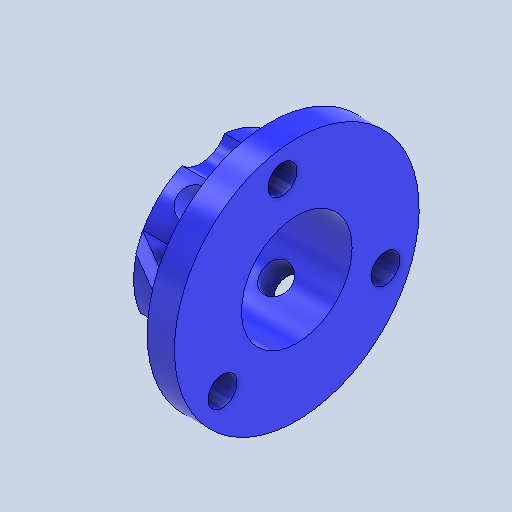
# Autodesk Inventor part: install-encoder-v1-3DP-Shaft-F
Saved by Autodesk Inventor 2025.2 (Build 292293000, 293)
## iProperties
Created: 2024-02-12
Part Number: install-encoder-v1-3DP-Shaft-F
Material: ABS プラスチック
Document SubType Name: Modeling
Designer: haruy
Density: 1.06 g/cm^3
Appearance: 青 - 壁塗料 - 光沢
Author: haruy
Autodesk Inventor part; units mm, degrees
sketch "スケッチ1" plane through (0, 0, 0) normal (1, 0, 0) x (0, 1, 0)
  circle A0 centre (0, 0) radius 13.5
  circle A1 centre (0, 0) radius 6.1
  circle A2 centre (0, 0) radius 10.5
  circle A3 centre (10.3803, 1.5811) radius 1.6
  circle A4 centre (-6.5594, 8.199) radius 1.6
  circle A5 centre (-3.8208, -9.7801) radius 1.6
  circle A6 centre (0, 0) radius 9
  circle A7 centre (-6.5594, 8.199) radius 3
  circle A8 centre (10.3803, 1.5811) radius 3
  circle A9 centre (-3.8208, -9.7801) radius 3
  line L0 (0, 0) -> (8.4336, -10.5416)
  line L1 (4.8067, -7.6089) -> (7.6295, -11.1373)
  line L2 (6.3684, -6.3595) -> (9.1913, -9.8879)
  line L3 (0, 0) -> (10.3803, 1.5811)
  line L4 (0, 0) -> (-2.0329, 13.3461)
  line L5 (0, 0) -> (-3.8208, -9.7801)
  line L6 (0, 0) -> (-12.5745, 4.9125)
  point P0 (-5.3784, -7.2162)
  point P1 (-0.9377, -8.951)
  point P2 (8.9386, -1.0497)
  point P3 (8.2206, 3.6635)
  point P4 (-3.5602, 8.2659)
  point P5 (-7.283, 5.2876)
  dimension "d2" = 21
  dimension "d0" = 27
  dimension "d1" = 12.2
  dimension "d3" = 3.2
  dimension "d6" = 360
  dimension "d10" = 18
  dimension "d11" = 6
  dimension "d12" = 6
  dimension "d13" = 6
  dimension "d17" = 60
  dimension "d18" = 1
  dimension "d19" = 1
  dimension "d32" = 90
  dimension "d33" = 90
  constraints: 14 end point, 9 centre point, 7 coincident, 7 point on circle, 2 parallel, 10 other
  measures "d0" diameter of A0
  measures "d1" diameter of A1
  measures "d3" diameter of A3
  measures "d10" diameter of A6
  measures "d11" diameter of A7
  measures "d12" diameter of A8
  measures "d13" diameter of A9
  measures "d18" distance between parallel lines of L0 L2
  measures "d19" distance between parallel lines of L0 L1
extrude "押し出し1" add sketch "スケッチ1" along normal blind 3 contours L1 A2 L0 A0 | A0 A9 A2 L1 | L0 A2 L2 A0 | A0 L6 A2 A9 | A9 A2 A5 | L1 A6 L0 A2 | A2 A9 A6 L1 | L2 A2 A8 A0 | L0 A6 L2 A2 | A0 A7 A2 L6 | A9 A6 A5 A2 | A2 L6 A6 A9 | A2 A5 A6 A9 | A6 A9 L5 A1 L0 | L2 A6 A8 A2 | L0 A1 L3 A8 A6 | A0 L4 A2 A7 | A7 A2 A4 | A2 A7 A6 L6 | A9 L5 A5 A6 | A6 L6 A1 L5 A9 | A6 A5 L5 A9 | A8 A2 L4 A0 | A8 A2 A3 | A8 A6 A3 A2 | A7 A6 A4 A2 | A2 L4 A6 A7 | A2 A4 A6 A7 | A6 A7 L4 A1 L6 | A8 A6 L4 A2 | A2 A3 A6 A8 | A8 L3 A3 A6 | A7 A6 A4 | A8 L3 A1 L4 A6 | A6 A3 L3 A8
extrude "押し出し2" add sketch "スケッチ1" against normal blind 6 contours A6 A9 L5 A1 L0 | L0 A1 L3 A8 A6 | A6 L6 A1 L5 A9 | A6 A7 L4 A1 L6 | A8 L3 A1 L4 A6
extrude "押し出し4" add sketch "スケッチ1" against normal up to surface (6 mm away) contours L1 A2 L0 A0 | L0 A2 L2 A0 | L1 A6 L0 A2 | L0 A6 L2 A2
ref_plane "作業平面1" through (-6, 8.4104, -10.5126) normal (0, -0.7808577, -0.624709) x (1, 0, 0)
sketch "スケッチ3" plane through (-6, 8.4104, -10.5126) normal (0, -0.7808577, -0.624709) x (1, 0, 0)
  line L0 (0, -0.0371) -> (9, -0.0371) projected
  line L1 (6, -0.0371) -> (0, -0.0371)
  line L2 (0, -0.0371) -> (0, 4.4629)
  line L3 (0, 4.4629) -> (6, 4.4629)
  line L4 (6, 4.4629) -> (6, -0.0371)
  line L5 (0, 4.4629) -> (6, -0.0371)
  point P0 (6, 13.4629)
  dimension "d28" = 6
  dimension "d29" = 4.5
  constraints: 10 end point, 2 parallel, 1 horizontal, 1 perpendicular, 1 point on line
  measures "d28" distance of L2.end L3.end
  measures "d29" distance of L1.end L2.end
extrude "押し出し5" cut sketch "スケッチ3" along normal through all both and the other way through all contours L2 L5 L0
ref_plane "作業平面3" through (0, 0, 0) normal (0, -0.150585, 0.9885971) x (1, 0, 0)
mirror "ミラー1" about plane through (0, 0, 0) normal (0, -0.150585, 0.9885971) of "押し出し5", "押し出し4"
ref_plane "作業平面4" through (0, 0, 0) normal (0, -0.9314427, 0.3638881) x (1, 0, 0)
mirror "ミラー2" about plane through (0, 0, 0) normal (0, -0.9314427, 0.3638881) of "押し出し5", "押し出し4"
sketch "スケッチ4" plane through (-6, 0, 0) normal (-1, 0, 0) x (0, 0, 1)
  arc A0 (-7.2162, -5.3784) -> (-2.3355, -8.6917) centre (0, 0) ccw projected
  arc A1 (-7.2162, -5.3784) -> (-2.3355, -8.6917) centre (0, 0) ccw projected
  point P0 (-7.2162, -5.3784)
  point P1 (-5.5459, -7.0882)
  dimension "d35" = 23
  constraints: 2 coincident, 1 point on circle
ref_plane "作業平面5" through (-6, -7.0882, -5.5459) normal (0, -0.7875786, -0.6162142) x (1, 0, 0)
sketch "スケッチ5" plane through (-6, -7.0882, -5.5459) normal (0, -0.7875786, -0.6162142) x (1, 0, 0)
  line L0 (0, 3.5166) -> (0, -2.3691) projected
  point P0 (6, 0)
  point P1 (3, 0)
  point P2 (0, 0.5738)
  dimension "d36" = 3
  constraints: 1 midpoint
  measures "d36" horizontal distance of point (3, 0) point (0, 0.574)
hole "穴1" at (-3, -7.0882, -5.5459) direction (0, 0.7875786, 0.6162142) diameter 3.2 end through all
